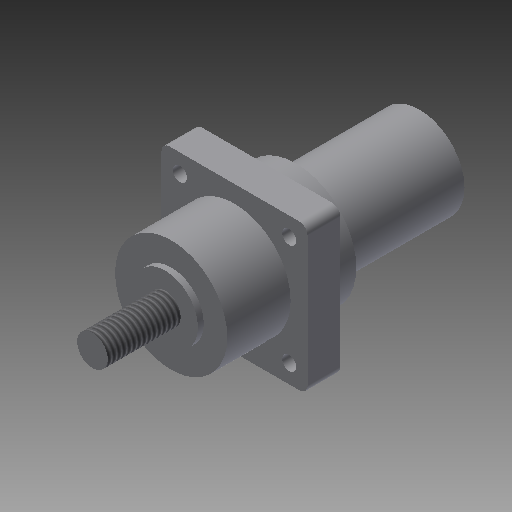
# Autodesk Inventor part: Pg_15
Saved by Autodesk Inventor 2017 (Build 210142000, 142)
## iProperties
Created: 2013-03-10
Part Number: Pg_15
Material: Generic
Document SubType Name: Modeling
Designer: user
Density: 1 g/cm^3
Mass: 146.717 g
Surface Area: 215.379 cm^2
Volume: 146.717 cm^3
Appearance: Default
Author: user
Autodesk Inventor part; units mm, degrees
ref_plane "YZ Plane" through (0, 0, 0) normal (1, 0, 0) x (0, 1, 0)
ref_plane "XZ Plane" through (0, 0, 0) normal (0, 1, 0) x (-1, 0, 0)
ref_plane "XY Plane" through (0, 0, 0) normal (0, 0, 1) x (1, 0, 0)
sketch "Sketch1" plane through (0, 0, 0) normal (0, 0, 1) x (1, 0, 0)
  line L0 (-28.448, 28.448) -> (28.448, 28.448)
  line L1 (28.448, 28.448) -> (28.448, -28.448)
  line L2 (28.448, -28.448) -> (-28.448, -28.448)
  line L3 (-28.448, -28.448) -> (-28.448, 28.448)
  point P0 (0, 0)
  point P1 (-28.448, 0)
  point P2 (0, 28.448)
  dimension "d0" = 56.896
  constraints: 8 end point, 2 midpoint, 2 parallel, 2 perpendicular, 1 horizontal, 1 horizontal alignment, 1 vertical alignment
  measures "d0" distance of L0.start L0.end
extrude "Extrusion1" add sketch "Sketch1" along normal blind 12.7
sketch "Sketch2" plane through (0, 0, 12.7) normal (0, 0, 1) x (1, 0, 0)
  circle A0 centre (0, 0) radius 21.844
  dimension "d4" = 43.688
  constraints: 1 centre point, 1 coincident
  measures "d4" diameter of A0
extrude "Extrusion2" add sketch "Sketch2" along normal blind 24.638
sketch "Sketch3" plane through (0, 0, 37.338) normal (0, 0, 1) x (1, 0, 0)
  circle A0 centre (0, 0) radius 21.844 projected
  circle A1 centre (0, 0) radius 6
  dimension "d8" = 12
  constraints: 1 centre point, 1 coincident
  measures "d8" diameter of A1
extrude "Extrusion3" add sketch "Sketch3" along normal blind 30.64 contours A1
thread "Thread1" size "1/2-13 UNC" class "2A" standard "ANSI Unified Screw Threads" full length
sketch "Sketch4" plane through (0, 0, 0) normal (0, 0, -1) x (-1, 0, 0)
  circle A0 centre (0, 0) radius 23.425
  dimension "d14" = 46.85
  constraints: 1 centre point, 1 coincident
  measures "d14" diameter of A0
extrude "Extrusion4" add sketch "Sketch4" along normal blind 11.25
fillet "Fillet1" radius 3.175 4 edges at (28.448, 28.448, 6.35) (-28.448, 28.448, 6.35) (28.448, -28.448, 6.35) (-28.448, -28.448, 6.35)
sketch "Sketch5" plane through (0, 0, -11.25) normal (0, 0, -1) x (-1, 0, 0)
  circle A0 centre (0, 0) radius 23.425 projected
  circle A1 centre (0, 0) radius 17.5
  dimension "d21" = 35
  constraints: 1 centre point, 1 coincident
  measures "d21" diameter of A1
extrude "Extrusion5" add sketch "Sketch5" along normal blind 48.05 contours A1
sketch "Sketch6" plane through (0, 0, 12.7) normal (0, 0, 1) x (1, 0, 0)
  line L0 (28.448, -25.273) -> (28.448, 25.273) projected
  line L1 (25.273, 28.448) -> (-25.273, 28.448) projected
  line L2 (-28.448, 25.273) -> (-28.448, -25.273) projected
  line L3 (21.2598, 21.2598) -> (21.2598, -21.2598)
  line L4 (-21.2598, 21.2598) -> (21.2598, 21.2598)
  point P0 (-21.2598, -21.2598)
  point P1 (0, 21.2598)
  point P2 (0, 28.448)
  point P3 (21.2598, 0)
  point P4 (28.448, 0)
  dimension "d25" = 42.5196
  dimension "d27" = 42.5196
  constraints: 4 end point, 4 midpoint, 3 horizontal alignment, 3 vertical alignment, 1 parallel, 1 perpendicular
  measures "d25" distance of L3.start L4.start
  measures "d27" distance of L3.end L3.start
hole "Hole1" at (-21.2598, 21.2598, 12.7) at (21.2598, 21.2598, 12.7) at (21.2598, -21.2598, 12.7) at (-21.2598, -21.2598, 12.7) direction (0, 0, -1) diameter 5.5 end through all
sketch "Sketch7" plane through (0, 0, 37.338) normal (0, 0, 1) x (1, 0, 0)
  circle A0 centre (0, 0) radius 6 projected
  circle A1 centre (0, 0) radius 21.844 projected
  circle A2 centre (0, 0) radius 12.7
  dimension "d35" = 25.4
  constraints: 1 centre point, 1 coincident
  measures "d35" diameter of A2
extrude "Extrusion6" add sketch "Sketch7" along normal blind 2.286 contours A2
body "Solid1"
